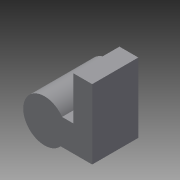
# Autodesk Inventor part: goal holder flipped
Saved by Autodesk Inventor 2015 (Build 190159000, 159)
## iProperties
Created: 2014-11-06
Part Number: goal holder flipped
Material: Generic
Document SubType Name: Modeling
Designer: jesse
Density: 1 g/cm^3
Appearance: Default
Author: jesse
Autodesk Inventor part; units mm, degrees
ref_plane "YZ Plane" through (0, 0, 0) normal (1, 0, 0) x (0, 1, 0)
ref_plane "XZ Plane" through (0, 0, 0) normal (0, 1, 0) x (-1, 0, 0)
ref_plane "XY Plane" through (0, 0, 0) normal (0, 0, 1) x (1, 0, 0)
sketch "Sketch1" plane through (0, 0, 0) normal (0, 0, 1) x (1, 0, 0)
  circle A0 centre (0, 0) radius 11 projected
  circle A1 centre (0, 0) radius 1.75 projected
  circle A2 centre (-8, 0) radius 1.75 projected
  circle A3 centre (0, 8) radius 1.75 projected
  circle A4 centre (8, 0) radius 1.75 projected
  circle A5 centre (0, -8) radius 1.75 projected
extrude "Extrusion1" add sketch "Sketch1" along normal blind 9.525
sketch "Sketch2" plane through (0, 0, 9.525) normal (0, 0, 1) x (1, 0, 0)
  circle A0 centre (0, 0) radius 11 projected
  line L0 (9.0377, 6.2705) -> (14.8574, 6.2705)
  line L1 (14.8574, 6.2705) -> (14.8574, 19.7717)
  line L2 (22.8575, 28.6861) -> (24.5877, 28.6861)
  line L3 (24.5877, 28.6861) -> (24.5877, -7.2164)
  line L4 (24.5877, -7.2164) -> (8.302, -7.2164)
  line L5 (22.8575, 28.6861) -> (14.8574, 28.6861)
  line L6 (14.8574, 19.7717) -> (14.8574, 28.6861)
  point P0 (-11, -11)
  constraints: 14 end point, 3 perpendicular, 2 point on circle, 1 horizontal, 1 parallel, 1 vertical
extrude "Extrusion2" add sketch "Sketch2" along normal blind 23.8125
body "Solid1"
